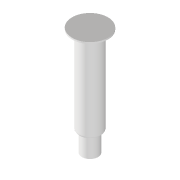
# Autodesk Inventor part: 00_5ml_glue_cartridge
Saved by Autodesk Inventor 2022 (Build 260153000, 153)
## iProperties
Created: 2022-08-23
Part Number: 00_5ml_glue_cartridge
Material: Generisch
Document SubType Name: Modeling
Designer: UC2
Density: 1 g/cm^3
Appearance: Rot
Author: UC2
Autodesk Inventor part; units mm, degrees
ref_plane "YZ Plane" through (0, 0, 0) normal (1, 0, 0) x (0, 1, 0)
ref_plane "XZ Plane" through (0, 0, 0) normal (0, 1, 0) x (-1, 0, 0)
ref_plane "XY Plane" through (0, 0, 0) normal (0, 0, 1) x (1, 0, 0)
sketch "Skizze1" plane through (0, 0, 0) normal (0, 0, 1) x (1, 0, 0)
  line L0 (0, 0) -> (5.15, 0)
  line L1 (5.15, 0) -> (5.15, 12)
  line L2 (0, 0) -> (0, 68.3)
  line L3 (0, 68.3) -> (7.15, 68.3)
  line L4 (7.15, 68.3) -> (7.15, 14)
  line L5 (5.15, 12) -> (5.15, 12)
  arc A0 (5.15, 12) -> (7.15, 14) centre (5.15, 14) ccw
  line L6 (7.15, 68.3) -> (11.4441, 68.3)
  line L7 (11.4441, 68.3) -> (11.4441, 69.3)
  line L8 (11.4441, 69.3) -> (0, 69.3)
  line L9 (0, 69.3) -> (0, 68.3)
  dimension "d0" = 5.15
  dimension "d1" = 12
  dimension "d2" = 68.3
  dimension "d3" = 7.15
  dimension "d4" = 2
  dimension "d5" = 1
  constraints: 20 end point, 4 perpendicular, 3 horizontal, 2 point on circle, 2 tangent, 2 vertical, 1 centre point, 1 parallel
  measures "d0" distance of L0.start L0.end
  measures "d1" distance of L0.end L1.end
  measures "d2" distance of L0.start L2.end
  measures "d3" distance of L2.end L3.end
  measures "d4" radius of A0
  measures "d5" distance of L6.end L7.end
revolve "Umdrehung1" add sketch "Skizze1" angle 360 about axis through (0, 0, 0) along (0, 1, 0)
